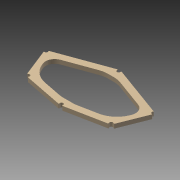
# Autodesk Inventor part: section1
Saved by Autodesk Inventor 2015 (Build 190159000, 159)
## iProperties
Created: 2017-09-23
Part Number: section1
Material: Polyethylene, High Density
Document SubType Name: Modeling
Designer: Mimoja
Density: 0.952 g/cm^3
Appearance: Smooth - Off-White
Mass: 523.935 g
Surface Area: 1008.07 cm^2
Volume: 550.352 cm^3
Author: Mimoja
Autodesk Inventor part; units mm, degrees
ref_plane "YZ Plane" through (0, 0, 0) normal (1, 0, 0) x (0, 1, 0)
ref_plane "XZ Plane" through (0, 0, 0) normal (0, 1, 0) x (-1, 0, 0)
ref_plane "XY Plane" through (0, 0, 0) normal (0, 0, 1) x (1, 0, 0)
sketch "Sketch1" plane through (0, 0, 0) normal (0, 0, 1) x (1, 0, 0)
  line L0 (0, 9.7536) -> (-185.3184, 46.3296)
  line L1 (-185.3184, 46.3296) -> (-240.1824, 184.7088)
  line L2 (-240.1824, 184.7088) -> (0, 272.1864)
  line L3 (0, 562.8605) -> (0, -145.2705) construction
  line L4 (0, 272.1864) -> (0, 9.7536)
  point P0 (0, 0)
  dimension "d9" = 272.1864
  dimension "d11" = 240.1824
  dimension "d15" = 184.7088
  dimension "d20" = 185.3184
  dimension "d22" = 46.3296
  dimension "d39" = 0
  dimension "d41" = 0
  dimension "d42" = 9.7536
  constraints: 10 end point, 1 vertical
  measures "d9" distance of point (0, 0) L2.end
  measures "d11" horizontal distance of point (0, 0) L1.end
  measures "d15" vertical distance of point (0, 0) L1.end
  measures "d20" horizontal distance of point (0, 0) L0.end
  measures "d22" vertical distance of point (0, 0) L0.end
  measures "d39" horizontal distance of point (0, 0) L2.end
  measures "d41" horizontal distance of point (0, 0) L0.start
  measures "d42" distance of point (0, 0) L0.start
extrude "Extrusion4" add sketch "Sketch1" along normal blind 18
hole "Hole2" at (0.0182, 265.1521, 18) direction (0, 0, -1) diameter 15 end through all
hole "Hole3" at (-233.7862, 182.8308, 18) direction (0, 0, -1) diameter 15 end through all
hole "Hole4" at (-180.9047, 51.7876, 18) direction (0, 0, -1) diameter 15 end through all
hole "Hole5" at (0.2097, 16.6506, 18) direction (0, 0, -1) diameter 15 end through all
sketch "Sketch6" plane through (0, 0, 18) normal (0, 0, 1) x (1, 0, 0)
  line L0 (-30, 231.4607) -> (-208.2387, 166.5438)
  line L1 (-208.2387, 166.5438) -> (-170.7523, 71.9949)
  line L2 (-170.7523, 71.9949) -> (-30, 44.2148)
  line L3 (-5.5654, 270.1594) -> (-229.1506, 188.7267) projected
  line L4 (-236.6974, 175.9189) -> (-188.1895, 53.5712) projected
  line L5 (-177.9802, 44.8813) -> (-4.1975, 10.582) projected
  line L6 (0, 231.4607) -> (-30, 231.4607)
  line L7 (0, 44.2148) -> (-30, 44.2148)
  line L8 (0, 44.2148) -> (0, 231.4607)
  point P0 (0, 0)
  dimension "d167" = 23
  dimension "d168" = 28
  dimension "d170" = 28
  dimension "d171" = 30
  dimension "d173" = 0
  dimension "d174" = 30
  constraints: 12 end point, 3 parallel, 2 horizontal, 1 vertical
  measures "d167" distance between parallel lines of L4 L1
  measures "d168" distance between parallel lines of L5 L2
  measures "d170" distance between parallel lines of L3 L0
  measures "d171" distance of L6.start L0.start
  measures "d173" distance from line of L8 point (0, 0)
  measures "d174" distance of L7.start L2.end
extrude "Extrusion6" cut sketch "Sketch6" against normal through all
fillet "Fillet6" radius 40 1 edges at (-208.2387, 166.5438, 9)
fillet "Fillet7" radius 100 1 edges at (-170.7523, 71.9949, 9)
fillet "Fillet8" radius 100 1 edges at (-30, 44.2148, 9)
fillet "Fillet9" radius 100 1 edges at (-30, 231.4607, 9)
fillet "Fillet10" radius 1.5 1 edges at (-5.5654, 270.1594, 9)
fillet "Fillet11" radius 1 1 edges at (-229.1506, 188.7267, 9)
fillet "Fillet12" radius 1 1 edges at (-236.6974, 175.9189, 9)
fillet "Fillet13" radius 2 1 edges at (-177.9802, 44.8813, 9)
fillet "Fillet14" radius 2 1 edges at (-188.1895, 53.5712, 9)
fillet "Fillet15" radius 2 1 edges at (-4.1975, 10.582, 9)
mirror "Mirror3" about plane through (0, 0, 0) normal (1, 0, 0)
body "Solid4"
